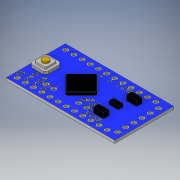
# Autodesk Inventor part: Arduino Pro Mini
Saved by Autodesk Inventor 2016 (Build 200138000, 138)
## iProperties
Created: 2015-11-30
Part Number: Arduino Pro Mini
Material: Generic
Document SubType Name: Modeling
Designer: Spooner
Density: 1 g/cm^3
Appearance: Default
Author: Spooner
Autodesk Inventor part; units mm, degrees
(part 1 of 2)
ref_plane "YZ Plane" through (0, 0, 0) normal (1, 0, 0) x (0, 1, 0)
ref_plane "XZ Plane" through (0, 0, 0) normal (0, 1, 0) x (-1, 0, 0)
sketch "Sketch1" plane through (0, 0, 0) normal (0, 1, 0) x (-1, 0, 0)
  line L0 (0, 0) -> (-33.6804, 0)
  line L1 (-33.6804, 0) -> (-33.6804, -18.3515)
  line L2 (-33.6804, -18.3515) -> (0, -18.3515)
  line L3 (0, -18.3515) -> (0, 0)
  dimension "d0" = 18.3515
  dimension "d1" = 33.6804
  constraints: 8 end point, 2 parallel, 1 horizontal, 1 perpendicular
  measures "d0" distance of L2.end L0.start
  measures "d1" distance of L0.start L0.end
extrude "Extrusion1" add sketch "Sketch1" along normal blind 0.8636
sketch "Sketch2" plane through (0, 0.8636, 0) normal (0, 1, 0) x (1, 0, 0)
  line L0 (14.0415, 4.3942) -> (18.9357, 9.2884)
  line L1 (18.9357, 9.2884) -> (14.0415, 14.1827)
  line L2 (14.0415, 14.1827) -> (9.1472, 9.2884)
  line L3 (9.1472, 9.2884) -> (14.0415, 4.3942)
  line L4 (14.0415, 4.3942) -> (14.0415, 14.1827) construction
  line L5 (18.9357, 9.2884) -> (9.1472, 9.2884) construction
  line L6 (0, 0) -> (33.6804, 0) projected
  line L7 (33.6804, 0) -> (33.6804, 18.3515) projected
  point P0 (14.0415, 9.2884)
  dimension "d4" = 6.9215
  dimension "d5" = 4.3942
  dimension "d6" = 45
  dimension "d7" = 14.7447
  constraints: 12 end point, 2 midpoint, 2 parallel, 2 perpendicular
  measures "d4" distance of L0.end L1.end
  measures "d5" distance from line of L0.start L6
  measures "d6" angle of L6 L0
  measures "d7" distance from line of L0.end L7
extrude "Extrusion2" add sketch "Sketch2" along normal blind 1.1049
chamfer "Chamfer1" distance 0.381 angle 45 4 edges at (14.0415, 1.4161, -4.3942) (18.9357, 1.4161, -9.2884) (14.0415, 1.4161, -14.1827) (9.1472, 1.4161, -9.2884)
chamfer "Chamfer2" distance 0.1905 angle 45 4 edges at (11.5943, 1.9685, -11.7356) (16.4886, 1.9685, -11.7356) (16.4886, 1.9685, -6.8413) (11.5943, 1.9685, -6.8413)
sketch "Sketch3" plane through (0, 0.8636, 0) normal (0, 1, 0) x (1, 0, 0)
  line L0 (0.508, 11.7157) -> (5.588, 11.7157)
  line L1 (5.588, 11.7157) -> (5.588, 6.6357)
  line L2 (5.588, 6.6357) -> (0.508, 6.6357)
  line L3 (0.508, 6.6357) -> (0.508, 11.7157)
  line L4 (0, 18.3515) -> (0, 0) projected
  point P0 (0.508, 9.1758)
  point P1 (0, 9.1758)
  dimension "d16" = 5.08
  dimension "d17" = 0.508
  constraints: 8 end point, 2 midpoint, 2 parallel, 2 perpendicular, 1 horizontal, 1 horizontal alignment
  measures "d16" distance of L0.start L0.end
  measures "d17" distance between parallel lines of L4 L3
extrude "Extrusion3" add sketch "Sketch3" along normal blind 0.889
chamfer "Chamfer3" distance 0.762 angle 45 4 edges at (5.588, 1.3081, -6.6357) (5.588, 1.3081, -11.7157) (0.508, 1.3081, -6.6357) (0.508, 1.3081, -11.7157)
sketch "Sketch4" plane through (0, 1.7526, 0) normal (0, 1, 0) x (1, 0, 0)
  line L0 (0.508, 10.9537) -> (1.27, 11.7157) projected
  line L1 (0.508, 10.9537) -> (0.508, 7.3978) projected
  line L2 (1.27, 6.6357) -> (0.508, 7.3978) projected
  line L3 (1.27, 6.6357) -> (4.826, 6.6357) projected
  line L4 (5.588, 7.3978) -> (4.826, 6.6357) projected
  line L5 (5.588, 7.3978) -> (5.588, 10.9537) projected
  line L6 (4.826, 11.7157) -> (5.588, 10.9537) projected
  line L7 (4.826, 11.7157) -> (1.27, 11.7157) projected
  line L8 (1.5856, 10.9537) -> (1.27, 10.6381)
  line L9 (1.27, 10.6381) -> (1.27, 7.7134)
  line L10 (1.27, 7.7134) -> (1.5856, 7.3978)
  line L11 (1.5856, 7.3978) -> (4.5104, 7.3978)
  line L12 (4.5104, 7.3978) -> (4.826, 7.7134)
  line L13 (4.826, 7.7134) -> (4.826, 10.6381)
  line L14 (4.826, 10.6381) -> (4.5104, 10.9537)
  line L15 (4.5104, 10.9537) -> (1.5856, 10.9537)
  point P0 (0, 0)
  dimension "d23" = 0.762
  constraints: 16 end point, 7 other
  measures "d23" distance between parallel lines of L5 L13
extrude "Extrusion4" add sketch "Sketch4" along normal blind 0.508 draft -5 contours L15 L14 L13 L12 L11 L10 L9 L8
sketch "Sketch5" plane through (0, 2.2606, 0) normal (0, 1, 0) x (1, 0, 0)
  circle A0 centre (3.048, 9.1758) radius 1.016
  line L0 (1.604, 10.9093) -> (4.492, 10.9093) projected
  line L1 (1.3144, 7.7318) -> (1.3144, 10.6197) projected
  point P0 (0, 0)
  point P1 (3.048, 10.9093)
  point P2 (1.3144, 9.1758)
  dimension "d26" = 2.032
  constraints: 2 midpoint, 1 centre point, 1 horizontal alignment, 1 vertical alignment
  measures "d26" diameter of A0
extrude "Extrusion5" add sketch "Sketch5" along normal blind 0.508
sketch "Sketch6" plane through (0, 0.8636, 0) normal (0, 1, 0) x (1, 0, 0)
  line L0 (24.8412, 14.1478) -> (28.0289, 14.1478)
  line L1 (28.0289, 14.1478) -> (28.0289, 12.4841)
  line L2 (28.0289, 12.4841) -> (24.8412, 12.4841)
  line L3 (24.8412, 12.4841) -> (24.8412, 14.1478)
  line L4 (22.9997, 5.7277) -> (26.1874, 5.7277)
  line L5 (26.1874, 5.7277) -> (26.1874, 4.064)
  line L6 (26.1874, 4.064) -> (22.9997, 4.064)
  line L7 (22.9997, 4.064) -> (22.9997, 5.7277)
  line L8 (33.6804, 0) -> (33.6804, 18.3515) projected
  line L9 (0, 0) -> (33.6804, 0) projected
  line L10 (33.6804, 18.3515) -> (0, 18.3515) projected
  dimension "d29" = 3.1877
  dimension "d30" = 1.6637
  dimension "d31" = 5.6515
  dimension "d32" = 7.493
  dimension "d33" = 4.064
  dimension "d34" = 4.2037
  constraints: 16 end point, 6 parallel, 2 horizontal, 2 perpendicular
  measures "d29" distance of L0.start L0.end
  measures "d30" distance of L0.end L1.end
  measures "d31" distance between parallel lines of L8 L1
  measures "d32" distance between parallel lines of L8 L5
  measures "d33" distance between parallel lines of L9 L6
  measures "d34" distance between parallel lines of L10 L0
extrude "Extrusion6" add sketch "Sketch6" along normal blind 1.6129
sketch "Sketch7" plane through (0, 0.8636, 0) normal (0, 1, 0) x (1, 0, 0)
  line L0 (23.1394, 10.2235) -> (26.0604, 10.2235)
  line L1 (26.0604, 10.2235) -> (26.0604, 8.7503)
  line L2 (26.0604, 8.7503) -> (23.1394, 8.7503)
  line L3 (23.1394, 8.7503) -> (23.1394, 10.2235)
  line L4 (33.6804, 0) -> (33.6804, 18.3515) projected
  line L5 (33.6804, 18.3515) -> (0, 18.3515) projected
  point P0 (0, 0)
  dimension "d37" = 2.921
  dimension "d38" = 1.4732
  dimension "d39" = 7.62
  dimension "d40" = 8.128
  constraints: 8 end point, 2 parallel, 1 horizontal, 1 perpendicular
  measures "d37" distance of L0.start L0.end
  measures "d38" distance of L2.end L0.start
  measures "d39" distance between parallel lines of L4 L1
  measures "d40" distance between parallel lines of L5 L0
extrude "Extrusion7" add sketch "Sketch7" along normal blind 1.016
sketch "Sketch8" plane through (0, 0.8636, 0) normal (0, 1, 0) x (1, 0, 0)
  circle A0 centre (1.778, 1.651) radius 0.508
  line L0 (0, 0) -> (33.6804, 0) projected
  line L1 (0, 18.3515) -> (0, 0) projected
  dimension "d43" = 1.016
  dimension "d44" = 1.143
  dimension "d45" = 1.27
  constraints: 1 centre point
  measures "d43" diameter of A0
  measures "d44" distance edge to line of A0 L0
  measures "d45" distance edge to line of A0 L1
extrude "Extrusion8" cut sketch "Sketch8" against normal through all
sketch "Sketch9" plane through (0, 0.8636, 0) normal (0, 1, 0) x (1, 0, 0)
  circle A0 centre (1.778, 1.651) radius 0.508 projected
  circle A1 centre (1.778, 1.651) radius 0.762
  point P0 (0, 0)
  dimension "d48" = 1.524
  constraints: 1 centre point, 1 coincident
  measures "d48" diameter of A1
extrude "Extrusion9" add sketch "Sketch9" along normal blind 0.0254
pattern_linear "Rectangular Pattern1" count 12 spacing 2.54 along (1, 0, 0) of "Extrusion9", "Extrusion8"
sketch "Sketch10" plane through (0, 0.8636, 0) normal (0, 1, 0) x (1, 0, 0)
  circle A0 centre (31.9024, 2.667) radius 0.508
  circle A1 centre (1.778, 1.651) radius 0.508 projected
  line L0 (33.6804, 0) -> (33.6804, 18.3515) projected
  line L1 (0, 0) -> (33.6804, 0) projected
  dimension "d54" = 1.27
  dimension "d55" = 2.159
  constraints: 1 centre point, 1 equal radius
  measures "d54" distance edge to line of A0 L0
  measures "d55" distance edge to line of A0 L1
extrude "Extrusion10" cut sketch "Sketch10" against normal through all contours A0
sketch "Sketch11" plane through (0, 0.8636, 0) normal (0, 1, 0) x (1, 0, 0)
  circle A0 centre (1.778, 1.651) radius 0.762 projected
  circle A1 centre (31.9024, 2.667) radius 0.508 projected
  circle A2 centre (31.9024, 2.667) radius 0.762
  point P0 (0, 0)
  constraints: 1 centre point, 1 coincident, 1 equal radius
extrude "Extrusion11" add sketch "Sketch11" along normal blind 0.0254 contours A2
pattern_linear "Rectangular Pattern2" count 6 spacing 2.54 along (0, 0, -1) of "Extrusion11", "Extrusion10"
ref_plane "Work Plane1" through (0, 0, -9.1758) normal (0, 0, 1) x (1, 0, 0)
mirror "Mirror1" about plane through (0, 0, -9.1758) normal (0, 0, 1) of "Extrusion9", "Extrusion8", "Rectangular Pattern1"
sketch "Sketch12" plane through (0, 0.8636, 0) normal (0, 1, 0) x (1, 0, 0)
  circle A0 centre (7.8232, 4.445) radius 0.508
  circle A1 centre (18.034, 4.445) radius 0.508
  circle A2 centre (1.778, 1.651) radius 0.508 projected
  line L0 (0, 0) -> (33.6804, 0) projected
  line L1 (0, 18.3515) -> (0, 0) projected
  dimension "d63" = 3.937
  dimension "d64" = 7.3152
  dimension "d65" = 17.526
  constraints: 2 centre point, 2 equal radius, 1 horizontal alignment
  measures "d63" distance edge to line of A0 L0
  measures "d64" distance edge to line of A0 L1
  measures "d65" distance edge to line of A1 L1
extrude "Extrusion12" cut sketch "Sketch12" against normal through all contours A0 | A1
sketch "Sketch13" plane through (0, 0.8636, 0) normal (0, 1, 0) x (1, 0, 0)
  circle A0 centre (7.8232, 4.445) radius 0.762
  circle A1 centre (18.034, 4.445) radius 0.762
  circle A2 centre (18.034, 4.445) radius 0.508 projected
  circle A3 centre (7.8232, 4.445) radius 0.508 projected
  circle A4 centre (4.318, 1.651) radius 0.762 projected
  point P0 (0, 0)
  constraints: 2 centre point, 2 concentric, 2 equal radius
extrude "Extrusion13" add sketch "Sketch13" along normal blind 0.0254 contours A0 | A1
pattern_linear "Rectangular Pattern3" count 2 spacing 2.54 along (1, 0, 0) of "Extrusion12", "Extrusion13"
sketch "Sketch14" plane through (0, 0.8636, 0) normal (0, 1, 0) x (1, 0, 0)
  line L0 (0.4732, 2.286) -> (0.4732, 4.4742) construction
  line L1 (0.4732, 4.4742) -> (1.778, 4.4742) construction
  line L2 (1.778, 4.4742) -> (1.778, 2.286) construction
  line L3 (1.778, 2.286) -> (0.4732, 2.286) construction
  line L4 (0, 18.3515) -> (0, 0) projected
  circle A0 centre (1.778, 1.651) radius 0.508 projected
  line L5 (3.0132, 2.286) -> (3.0132, 4.4742) construction
  line L6 (3.0132, 4.4742) -> (4.318, 4.4742) construction
  line L7 (4.318, 4.4742) -> (4.318, 2.286) construction
  line L8 (4.318, 2.286) -> (3.0132, 2.286) construction
  circle A1 centre (4.318, 1.651) radius 0.508 projected
  line L9 (6.858, 2.286) -> (5.5532, 2.286) construction
  line L10 (5.5532, 2.286) -> (5.5532, 4.4742) construction
  line L11 (5.5532, 4.4742) -> (6.858, 4.4742) construction
  line L12 (6.858, 4.4742) -> (6.858, 2.286) construction
  circle A2 centre (6.858, 1.651) radius 0.508 projected
  line L13 (9.398, 2.286) -> (8.0932, 2.286) construction
  line L14 (8.0932, 2.286) -> (8.0932, 4.4742) construction
  line L15 (8.0932, 4.4742) -> (9.398, 4.4742) construction
  line L16 (9.398, 4.4742) -> (9.398, 2.286) construction
  circle A3 centre (9.398, 1.651) radius 0.508 projected
  line L17 (17.1114, 6.0026) -> (18.6587, 7.5499) construction
  line L18 (18.6587, 7.5499) -> (19.5813, 6.6273) construction
  line L19 (19.5813, 6.6273) -> (18.034, 5.08) construction
  line L20 (18.034, 5.08) -> (17.1114, 6.0026) construction
  line L21 (19.6514, 6.0026) -> (21.1987, 7.5499) construction
  line L22 (21.1987, 7.5499) -> (22.1213, 6.6273) construction
  line L23 (22.1213, 6.6273) -> (20.574, 5.08) construction
  line L24 (20.574, 5.08) -> (19.6514, 6.0026) construction
  circle A4 centre (18.034, 4.445) radius 0.508 projected
  circle A5 centre (20.574, 4.445) radius 0.508 projected
  line L25 (14.3109, 4.6636) -> (18.6663, 9.019) projected
  line L26 (22.6916, 2.286) -> (21.3868, 2.286) construction
  line L27 (21.3868, 2.286) -> (21.3868, 4.4742) construction
  line L28 (21.3868, 4.4742) -> (22.6916, 4.4742) construction
  line L29 (22.6916, 4.4742) -> (22.6916, 2.286) construction
  circle A6 centre (22.098, 1.651) radius 0.508 projected
  line L30 (22.905, 3.7002) -> (26.371, 3.7002) construction
  line L31 (26.371, 3.7002) -> (26.371, 2.4138) construction
  line L32 (26.371, 2.4138) -> (22.905, 2.4138) construction
  line L33 (22.905, 2.4138) -> (22.905, 3.7002) construction
  circle A7 centre (24.638, 1.651) radius 0.508 projected
  line L34 (20.365, 16.0655) -> (23.831, 16.0655) construction
  line L35 (23.831, 16.0655) -> (23.831, 14.7791) construction
  line L36 (23.831, 14.7791) -> (20.365, 14.7791) construction
  line L37 (20.365, 14.7791) -> (20.365, 16.0655) construction
  circle A8 centre (22.098, 16.7005) radius 0.508 projected
  circle A9 centre (19.558, 16.7005) radius 0.508 projected
  circle A10 centre (17.018, 16.7005) radius 0.508 projected
  circle A11 centre (14.478, 16.7005) radius 0.508 projected
  line L38 (17.825, 14.7791) -> (17.825, 16.0655) construction
  line L39 (17.825, 16.0655) -> (21.291, 16.0655) construction
  line L40 (21.291, 16.0655) -> (21.291, 14.7791) construction
  line L41 (21.291, 14.7791) -> (17.825, 14.7791) construction
  line L42 (15.4312, 14.7791) -> (15.4312, 16.0655) construction
  line L43 (15.4312, 16.0655) -> (18.6048, 16.0655) construction
  line L44 (18.6048, 16.0655) -> (18.6048, 14.7791) construction
  line L45 (18.6048, 14.7791) -> (15.4312, 14.7791) construction
  line L46 (12.745, 14.7791) -> (12.745, 16.0655) construction
  line L47 (12.745, 16.0655) -> (16.211, 16.0655) construction
  line L48 (16.211, 16.0655) -> (16.211, 14.7791) construction
  line L49 (16.211, 14.7791) -> (12.745, 14.7791) construction
  spline S0 degree 2 poles (1.576, 3.2573) (1.69, 3.1646) (1.778, 2.9877) (1.778, 2.863) knots 0 0 0 1 2 2 2
  spline S1 degree 2 poles (1.778, 2.863) (1.778, 2.6504) (1.5982, 2.516) knots 0 0 0 1 1 1
  spline S2 degree 2 poles (1.5982, 2.516) (1.4165, 2.3778) (1.1227, 2.3778) knots 0 0 0 1 1 1
  spline S3 degree 2 poles (1.1227, 2.3778) (0.798, 2.3778) (0.6278, 2.5334) knots 0 0 0 1 1 1
  spline S4 degree 2 poles (0.6278, 2.5334) (0.4916, 2.6581) (0.4916, 2.8379) knots 0 0 0 1 1 1
  spline S5 degree 2 poles (0.4916, 2.8379) (0.4916, 2.978) (0.5331, 3.0592) knots 0 0 0 1 1 1
  spline S6 degree 2 poles (0.5331, 3.0592) (0.5795, 3.1491) (0.6945, 3.2119) knots 0 0 0 1 1 1
  spline S7 degree 2 poles (0.6945, 3.2119) (0.7187, 3.2255) (0.7409, 3.2255) knots 0 0 0 1 1 1
  spline S8 degree 2 poles (0.7409, 3.2255) (0.7796, 3.2255) (0.8327, 3.1675) (0.8327, 3.1317) knots 0 0 0 1 2 2 2
  spline S9 degree 2 poles (0.8327, 3.1317) (0.8327, 3.0814) (0.7786, 3.0524) knots 0 0 0 1 1 1
  spline S10 degree 2 poles (0.7786, 3.0524) (0.7226, 3.0196) (0.6984, 2.9635) knots 0 0 0 1 1 1
  spline S11 degree 2 poles (0.6984, 2.9635) (0.6781, 2.921) (0.6781, 2.8369) knots 0 0 0 1 1 1
  spline S12 degree 2 poles (0.6781, 2.8369) (0.6781, 2.7277) (0.7757, 2.6523) knots 0 0 0 1 1 1
  spline S13 degree 2 poles (0.7757, 2.6523) (0.8936, 2.5595) (1.1227, 2.5595) knots 0 0 0 1 1 1
  spline S14 degree 2 poles (1.1227, 2.5595) (1.3334, 2.5595) (1.5915, 2.7345) (1.5915, 2.8659) knots 0 0 0 1 2 2 2
  spline S15 degree 2 poles (1.5915, 2.8659) (1.5915, 3.008) (1.4562, 3.1153) knots 0 0 0 1 1 1
  spline S16 degree 2 poles (1.4562, 3.1153) (1.4233, 3.1423) (1.4233, 3.1839) knots 0 0 0 1 1 1
  spline S17 degree 2 poles (1.4233, 3.1839) (1.4233, 3.2197) (1.4803, 3.2796) (1.518, 3.2796) knots 0 0 0 1 2 2 2
  spline S18 degree 2 poles (1.518, 3.2796) (1.5489, 3.2796) (1.576, 3.2573) knots 0 0 0 1 1 1
  spline S19 degree 2 poles (1.4117, 4.3698) (1.778, 4.3698) (1.778, 3.9175) knots 0 0 0 1 1 1
  spline S20 degree 2 poles (1.778, 3.9175) (1.778, 3.6459) (1.5064, 3.499) knots 0 0 0 1 1 1
  spline S21 degree 2 poles (1.5064, 3.499) (1.489, 3.4883) (1.4619, 3.4883) knots 0 0 0 1 1 1
  spline S22 degree 2 poles (1.4619, 3.4883) (1.4214, 3.4883) (1.3585, 3.5483) (1.3585, 3.5869) knots 0 0 0 1 2 2 2
  spline S23 degree 2 poles (1.3585, 3.5869) (1.3585, 3.6333) (1.4011, 3.6517) knots 0 0 0 1 1 1
  spline S24 degree 2 poles (1.4011, 3.6517) (1.5915, 3.7377) (1.5915, 3.9175) knots 0 0 0 1 1 1
  spline S25 degree 2 poles (1.5915, 3.9175) (1.5915, 4.1823) (1.4136, 4.1823) knots 0 0 0 1 1 1
  spline S26 degree 2 poles (1.4136, 4.1823) (1.3257, 4.1823) (1.2561, 4.0161) knots 0 0 0 1 1 1
  spline S27 degree 2 poles (1.2561, 4.0161) (1.1217, 3.6952) (1.1188, 3.6884) knots 0 0 0 1 1 1
  spline S28 degree 2 poles (1.1188, 3.6884) (1.0058, 3.499) (0.8192, 3.499) knots 0 0 0 1 1 1
  spline S29 degree 2 poles (0.8192, 3.499) (0.6452, 3.499) (0.5554, 3.6266) knots 0 0 0 1 1 1
  spline S30 degree 2 poles (0.5554, 3.6266) (0.4848, 3.728) (0.479, 3.8914) knots 0 0 0 1 1 1
  spline S31 degree 2 poles (0.479, 3.8914) (0.4732, 4.0422) (0.5515, 4.1639) knots 0 0 0 1 1 1
  spline S32 degree 2 poles (0.5515, 4.1639) (0.6153, 4.2761) (0.7467, 4.3176) knots 0 0 0 1 1 1
  spline S33 degree 2 poles (0.7467, 4.3176) (0.768, 4.3234) (0.7825, 4.3234) knots 0 0 0 1 1 1
  spline S34 degree 2 poles (0.7825, 4.3234) (0.8212, 4.3234) (0.8685, 4.2664) (0.8685, 4.2297) knots 0 0 0 1 2 2 2
  spline S35 degree 2 poles (0.8685, 4.2297) (0.8685, 4.162) (0.8163, 4.1456) knots 0 0 0 1 1 1
  spline S36 degree 2 poles (0.8163, 4.1456) (0.7371, 4.1204) (0.6578, 3.9822) (0.6617, 3.8981) knots 0 0 0 1 2 2 2
  spline S37 degree 2 poles (0.6617, 3.8981) (0.6704, 3.6807) (0.8154, 3.6807) knots 0 0 0 1 1 1
  spline S38 degree 2 poles (0.8154, 3.6807) (0.8917, 3.6807) (0.9449, 3.757) knots 0 0 0 1 1 1
  spline S39 degree 2 poles (0.9449, 3.757) (0.9855, 3.8141) (1.0348, 3.9503) knots 0 0 0 1 1 1
  spline S40 degree 2 poles (1.0348, 3.9503) (1.1092, 4.1572) (1.1585, 4.2287) knots 0 0 0 1 1 1
  spline S41 degree 2 poles (1.1585, 4.2287) (1.2561, 4.3698) (1.4117, 4.3698) knots 0 0 0 1 1 1
  spline S42 degree 2 poles (4.2155, 3.4178) (4.3093, 3.4178) (4.3093, 3.326) knots 0 0 0 1 1 1
  spline S43 degree 2 poles (4.3093, 3.326) (4.3093, 3.2342) (4.2155, 3.2342) knots 0 0 0 1 1 1
  line L50 (4.2155, 3.2342) -> (3.3621, 3.2342)
  line L51 (3.3621, 3.2342) -> (3.7439, 3.0003)
  spline S44 degree 2 poles (3.7439, 3.0003) (3.8028, 2.9587) (3.8028, 2.8988) knots 0 0 0 1 1 1
  spline S45 degree 2 poles (3.8028, 2.8988) (3.8028, 2.8408) (3.7487, 2.805) knots 0 0 0 1 1 1
  line L52 (3.7487, 2.805) -> (3.3534, 2.5731)
  line L53 (3.3534, 2.5731) -> (4.2155, 2.5731)
  spline S46 degree 2 poles (4.2155, 2.5731) (4.3093, 2.5731) (4.3093, 2.4812) knots 0 0 0 1 1 1
  spline S47 degree 2 poles (4.3093, 2.4812) (4.3093, 2.3875) (4.2155, 2.3875) knots 0 0 0 1 1 1
  line L54 (4.2155, 2.3875) -> (3.1466, 2.3875)
  spline S48 degree 2 poles (3.1466, 2.3875) (3.048, 2.3875) (3.048, 2.487) knots 0 0 0 1 1 1
  spline S49 degree 2 poles (3.048, 2.487) (3.048, 2.5557) (3.1031, 2.5943) knots 0 0 0 1 1 1
  line L55 (3.1031, 2.5943) -> (3.5612, 2.9017)
  line L56 (3.5612, 2.9017) -> (3.1128, 3.2052)
  spline S50 degree 2 poles (3.1128, 3.2052) (3.0393, 3.2564) (3.0393, 3.3221) knots 0 0 0 1 1 1
  spline S51 degree 2 poles (3.0393, 3.3221) (3.0393, 3.3627) (3.1012, 3.4178) (3.1466, 3.4178) knots 0 0 0 1 2 2 2
  line L57 (3.1466, 3.4178) -> (4.2155, 3.4178)
  spline S52 degree 2 poles (3.6801, 4.6491) (3.9353, 4.6491) (4.1015, 4.5293) knots 0 0 0 1 1 1
  spline S53 degree 2 poles (4.1015, 4.5293) (4.318, 4.3891) (4.318, 4.1736) knots 0 0 0 1 1 1
  spline S54 degree 2 poles (4.318, 4.1736) (4.318, 3.9571) (4.1179, 3.8189) knots 0 0 0 1 1 1
  spline S55 degree 2 poles (4.1179, 3.8189) (3.9343, 3.6903) (3.6801, 3.6903) knots 0 0 0 1 1 1
  spline S56 degree 2 poles (3.6801, 3.6903) (3.4259, 3.6903) (3.2394, 3.8112) knots 0 0 0 1 1 1
  spline S57 degree 2 poles (3.2394, 3.8112) (3.0316, 3.9445) (3.0316, 4.1533) knots 0 0 0 1 1 1
  spline S58 degree 2 poles (3.0316, 4.1533) (3.0316, 4.3766) (3.2384, 4.5206) knots 0 0 0 1 1 1
  spline S59 degree 2 poles (3.2384, 4.5206) (3.4259, 4.6491) (3.6801, 4.6491) knots 0 0 0 1 1 1
  spline S60 degree 2 poles (3.6801, 4.4655) (3.4945, 4.4655) (3.3554, 4.3843) knots 0 0 0 1 1 1
  spline S61 degree 2 poles (3.3554, 4.3843) (3.2181, 4.2992) (3.2181, 4.1533) knots 0 0 0 1 1 1
  spline S62 degree 2 poles (3.2181, 4.1533) (3.2181, 4.019) (3.3708, 3.9358) knots 0 0 0 1 1 1
  spline S63 degree 2 poles (3.3708, 3.9358) (3.4897, 3.874) (3.6801, 3.874) knots 0 0 0 1 1 1
  spline S64 degree 2 poles (3.6801, 3.874) (3.8666, 3.874) (3.9836, 3.931) knots 0 0 0 1 1 1
  spline S65 degree 2 poles (3.9836, 3.931) (4.1315, 4.0325) (4.1315, 4.1736) knots 0 0 0 1 1 1
  spline S66 degree 2 poles (4.1315, 4.1736) (4.1315, 4.3128) (3.9836, 4.3998) knots 0 0 0 1 1 1
  spline S67 degree 2 poles (3.9836, 4.3998) (3.8686, 4.4655) (3.6801, 4.4655) knots 0 0 0 1 1 1
  spline S68 degree 2 poles (3.9517, 5.7181) (4.318, 5.7181) (4.318, 5.2658) knots 0 0 0 1 1 1
  spline S69 degree 2 poles (4.318, 5.2658) (4.318, 4.9942) (4.0464, 4.8473) knots 0 0 0 1 1 1
  spline S70 degree 2 poles (4.0464, 4.8473) (4.029, 4.8366) (4.0019, 4.8366) knots 0 0 0 1 1 1
  spline S71 degree 2 poles (4.0019, 4.8366) (3.9614, 4.8366) (3.8985, 4.8966) (3.8985, 4.9352) knots 0 0 0 1 2 2 2
  spline S72 degree 2 poles (3.8985, 4.9352) (3.8985, 4.9816) (3.9411, 5) knots 0 0 0 1 1 1
  spline S73 degree 2 poles (3.9411, 5) (4.1315, 5.086) (4.1315, 5.2658) knots 0 0 0 1 1 1
  spline S74 degree 2 poles (4.1315, 5.2658) (4.1315, 5.5306) (3.9536, 5.5306) knots 0 0 0 1 1 1
  spline S75 degree 2 poles (3.9536, 5.5306) (3.8657, 5.5306) (3.7961, 5.3643) knots 0 0 0 1 1 1
  spline S76 degree 2 poles (3.7961, 5.3643) (3.6617, 5.0435) (3.6588, 5.0367) knots 0 0 0 1 1 1
  spline S77 degree 2 poles (3.6588, 5.0367) (3.5458, 4.8473) (3.3592, 4.8473) knots 0 0 0 1 1 1
  spline S78 degree 2 poles (3.3592, 4.8473) (3.1852, 4.8473) (3.0954, 4.9748) knots 0 0 0 1 1 1
  spline S79 degree 2 poles (3.0954, 4.9748) (3.0248, 5.0763) (3.019, 5.2397) knots 0 0 0 1 1 1
  spline S80 degree 2 poles (3.019, 5.2397) (3.0132, 5.3904) (3.0915, 5.5122) knots 0 0 0 1 1 1
  spline S81 degree 2 poles (3.0915, 5.5122) (3.1553, 5.6243) (3.2867, 5.6659) knots 0 0 0 1 1 1
  spline S82 degree 2 poles (3.2867, 5.6659) (3.308, 5.6717) (3.3225, 5.6717) knots 0 0 0 1 1 1
  spline S83 degree 2 poles (3.3225, 5.6717) (3.3612, 5.6717) (3.4085, 5.6147) (3.4085, 5.5779) knots 0 0 0 1 2 2 2
  spline S84 degree 2 poles (3.4085, 5.5779) (3.4085, 5.5103) (3.3563, 5.4939) knots 0 0 0 1 1 1
  spline S85 degree 2 poles (3.3563, 5.4939) (3.2771, 5.4687) (3.1978, 5.3305) (3.2017, 5.2464) knots 0 0 0 1 2 2 2
  spline S86 degree 2 poles (3.2017, 5.2464) (3.2104, 5.029) (3.3554, 5.029) knots 0 0 0 1 1 1
  spline S87 degree 2 poles (3.3554, 5.029) (3.4317, 5.029) (3.4849, 5.1053) knots 0 0 0 1 1 1
  spline S88 degree 2 poles (3.4849, 5.1053) (3.5255, 5.1623) (3.5748, 5.2986) knots 0 0 0 1 1 1
  spline S89 degree 2 poles (3.5748, 5.2986) (3.6492, 5.5055) (3.6985, 5.577) knots 0 0 0 1 1 1
  spline S90 degree 2 poles (3.6985, 5.577) (3.7961, 5.7181) (3.9517, 5.7181) knots 0 0 0 1 1 1
  spline S91 degree 2 poles (4.2136, 6.1453) (4.3093, 6.1453) (4.3093, 6.0535) knots 0 0 0 1 1 1
  spline S92 degree 2 poles (4.3093, 6.0535) (4.3093, 5.9617) (4.2136, 5.9617) knots 0 0 0 1 1 1
  line L58 (4.2136, 5.9617) -> (3.136, 5.9617)
  spline S93 degree 2 poles (3.136, 5.9617) (3.0432, 5.9617) (3.0432, 6.0535) knots 0 0 0 1 1 1
  spline S94 degree 2 poles (3.0432, 6.0535) (3.0432, 6.1453) (3.136, 6.1453) knots 0 0 0 1 1 1
  line L59 (3.136, 6.1453) -> (4.2136, 6.1453)
  spline S95 degree 2 poles (6.7555, 3.4178) (6.8493, 3.4178) (6.8493, 3.326) knots 0 0 0 1 1 1
  spline S96 degree 2 poles (6.8493, 3.326) (6.8493, 3.2342) (6.7555, 3.2342) knots 0 0 0 1 1 1
  line L60 (6.7555, 3.2342) -> (5.9021, 3.2342)
  line L61 (5.9021, 3.2342) -> (6.2839, 3.0003)
  spline S97 degree 2 poles (6.2839, 3.0003) (6.3428, 2.9587) (6.3428, 2.8988) knots 0 0 0 1 1 1
  spline S98 degree 2 poles (6.3428, 2.8988) (6.3428, 2.8408) (6.2887, 2.805) knots 0 0 0 1 1 1
  line L62 (6.2887, 2.805) -> (5.8934, 2.5731)
  line L63 (5.8934, 2.5731) -> (6.7555, 2.5731)
  spline S99 degree 2 poles (6.7555, 2.5731) (6.8493, 2.5731) (6.8493, 2.4812) knots 0 0 0 1 1 1
  spline S100 degree 2 poles (6.8493, 2.4812) (6.8493, 2.3875) (6.7555, 2.3875) knots 0 0 0 1 1 1
  line L64 (6.7555, 2.3875) -> (5.6866, 2.3875)
  spline S101 degree 2 poles (5.6866, 2.3875) (5.588, 2.3875) (5.588, 2.487) knots 0 0 0 1 1 1
  spline S102 degree 2 poles (5.588, 2.487) (5.588, 2.5557) (5.6431, 2.5943) knots 0 0 0 1 1 1
  line L65 (5.6431, 2.5943) -> (6.1012, 2.9017)
  line L66 (6.1012, 2.9017) -> (5.6528, 3.2052)
  spline S103 degree 2 poles (5.6528, 3.2052) (5.5793, 3.2564) (5.5793, 3.3221) knots 0 0 0 1 1 1
  spline S104 degree 2 poles (5.5793, 3.3221) (5.5793, 3.3627) (5.6412, 3.4178) (5.6866, 3.4178) knots 0 0 0 1 2 2 2
  line L67 (5.6866, 3.4178) -> (6.7555, 3.4178)
  spline S105 degree 2 poles (6.7536, 3.9155) (6.8493, 3.9155) (6.8493, 3.8237) knots 0 0 0 1 1 1
  spline S106 degree 2 poles (6.8493, 3.8237) (6.8493, 3.7319) (6.7536, 3.7319) knots 0 0 0 1 1 1
  line L68 (6.7536, 3.7319) -> (5.676, 3.7319)
  spline S107 degree 2 poles (5.676, 3.7319) (5.5832, 3.7319) (5.5832, 3.8237) knots 0 0 0 1 1 1
  spline S108 degree 2 poles (5.5832, 3.8237) (5.5832, 3.9155) (5.676, 3.9155) knots 0 0 0 1 1 1
  line L69 (5.676, 3.9155) -> (6.7536, 3.9155)
  spline S109 degree 2 poles (6.4917, 5.0986) (6.858, 5.0986) (6.858, 4.6462) knots 0 0 0 1 1 1
  spline S110 degree 2 poles (6.858, 4.6462) (6.858, 4.3746) (6.5864, 4.2277) knots 0 0 0 1 1 1
  spline S111 degree 2 poles (6.5864, 4.2277) (6.569, 4.2171) (6.5419, 4.2171) knots 0 0 0 1 1 1
  spline S112 degree 2 poles (6.5419, 4.2171) (6.5014, 4.2171) (6.4385, 4.277) (6.4385, 4.3157) knots 0 0 0 1 2 2 2
  spline S113 degree 2 poles (6.4385, 4.3157) (6.4385, 4.3621) (6.4811, 4.3804) knots 0 0 0 1 1 1
  spline S114 degree 2 poles (6.4811, 4.3804) (6.6715, 4.4665) (6.6715, 4.6462) knots 0 0 0 1 1 1
  spline S115 degree 2 poles (6.6715, 4.6462) (6.6715, 4.9111) (6.4936, 4.9111) knots 0 0 0 1 1 1
  spline S116 degree 2 poles (6.4936, 4.9111) (6.4057, 4.9111) (6.3361, 4.7448) knots 0 0 0 1 1 1
  spline S117 degree 2 poles (6.3361, 4.7448) (6.2017, 4.4239) (6.1988, 4.4172) knots 0 0 0 1 1 1
  spline S118 degree 2 poles (6.1988, 4.4172) (6.0858, 4.2277) (5.8992, 4.2277) knots 0 0 0 1 1 1
  spline S119 degree 2 poles (5.8992, 4.2277) (5.7252, 4.2277) (5.6354, 4.3553) knots 0 0 0 1 1 1
  spline S120 degree 2 poles (5.6354, 4.3553) (5.5648, 4.4568) (5.559, 4.6201) knots 0 0 0 1 1 1
  spline S121 degree 2 poles (5.559, 4.6201) (5.5532, 4.7709) (5.6315, 4.8927) knots 0 0 0 1 1 1
  spline S122 degree 2 poles (5.6315, 4.8927) (5.6953, 5.0048) (5.8267, 5.0464) knots 0 0 0 1 1 1
  spline S123 degree 2 poles (5.8267, 5.0464) (5.848, 5.0522) (5.8625, 5.0522) knots 0 0 0 1 1 1
  spline S124 degree 2 poles (5.8625, 5.0522) (5.9012, 5.0522) (5.9485, 4.9951) (5.9485, 4.9584) knots 0 0 0 1 2 2 2
  spline S125 degree 2 poles (5.9485, 4.9584) (5.9485, 4.8908) (5.8963, 4.8743) knots 0 0 0 1 1 1
  spline S126 degree 2 poles (5.8963, 4.8743) (5.8171, 4.8492) (5.7378, 4.711) (5.7417, 4.6269) knots 0 0 0 1 2 2 2
  spline S127 degree 2 poles (5.7417, 4.6269) (5.7504, 4.4094) (5.8954, 4.4094) knots 0 0 0 1 1 1
  spline S128 degree 2 poles (5.8954, 4.4094) (5.9717, 4.4094) (6.0249, 4.4858) knots 0 0 0 1 1 1
  spline S129 degree 2 poles (6.0249, 4.4858) (6.0655, 4.5428) (6.1148, 4.6791) knots 0 0 0 1 1 1
  spline S130 degree 2 poles (6.1148, 4.6791) (6.1892, 4.8859) (6.2385, 4.9574) knots 0 0 0 1 1 1
  spline S131 degree 2 poles (6.2385, 4.9574) (6.3361, 5.0986) (6.4917, 5.0986) knots 0 0 0 1 1 1
  spline S132 degree 2 poles (6.2201, 6.2593) (6.4753, 6.2593) (6.6415, 6.1395) knots 0 0 0 1 1 1
  spline S133 degree 2 poles (6.6415, 6.1395) (6.858, 5.9993) (6.858, 5.7838) knots 0 0 0 1 1 1
  spline S134 degree 2 poles (6.858, 5.7838) (6.858, 5.5673) (6.6579, 5.4291) knots 0 0 0 1 1 1
  spline S135 degree 2 poles (6.6579, 5.4291) (6.4743, 5.3006) (6.2201, 5.3006) knots 0 0 0 1 1 1
  spline S136 degree 2 poles (6.2201, 5.3006) (5.9659, 5.3006) (5.7794, 5.4214) knots 0 0 0 1 1 1
  spline S137 degree 2 poles (5.7794, 5.4214) (5.5716, 5.5548) (5.5716, 5.7635) knots 0 0 0 1 1 1
  spline S138 degree 2 poles (5.5716, 5.7635) (5.5716, 5.9868) (5.7784, 6.1308) knots 0 0 0 1 1 1
  spline S139 degree 2 poles (5.7784, 6.1308) (5.9659, 6.2593) (6.2201, 6.2593) knots 0 0 0 1 1 1
  spline S140 degree 2 poles (6.2201, 6.0757) (6.0345, 6.0757) (5.8954, 5.9945) knots 0 0 0 1 1 1
  spline S141 degree 2 poles (5.8954, 5.9945) (5.7581, 5.9095) (5.7581, 5.7635) knots 0 0 0 1 1 1
  spline S142 degree 2 poles (5.7581, 5.7635) (5.7581, 5.6292) (5.9108, 5.5461) knots 0 0 0 1 1 1
  spline S143 degree 2 poles (5.9108, 5.5461) (6.0297, 5.4842) (6.2201, 5.4842) knots 0 0 0 1 1 1
  spline S144 degree 2 poles (6.2201, 5.4842) (6.4066, 5.4842) (6.5236, 5.5412) knots 0 0 0 1 1 1
  spline S145 degree 2 poles (6.5236, 5.5412) (6.6715, 5.6427) (6.6715, 5.7838) knots 0 0 0 1 1 1
  spline S146 degree 2 poles (6.6715, 5.7838) (6.6715, 5.923) (6.5236, 6.01) knots 0 0 0 1 1 1
  spline S147 degree 2 poles (6.5236, 6.01) (6.4086, 6.0757) (6.2201, 6.0757) knots 0 0 0 1 1 1
  spline S148 degree 2 poles (9.0317, 3.2419) (9.398, 3.2419) (9.398, 2.7896) knots 0 0 0 1 1 1
  spline S149 degree 2 poles (9.398, 2.7896) (9.398, 2.518) (9.1264, 2.3711) knots 0 0 0 1 1 1
  spline S150 degree 2 poles (9.1264, 2.3711) (9.109, 2.3604) (9.0819, 2.3604) knots 0 0 0 1 1 1
  spline S151 degree 2 poles (9.0819, 2.3604) (9.0414, 2.3604) (8.9785, 2.4203) (8.9785, 2.459) knots 0 0 0 1 2 2 2
  spline S152 degree 2 poles (8.9785, 2.459) (8.9785, 2.5054) (9.0211, 2.5238) knots 0 0 0 1 1 1
  spline S153 degree 2 poles (9.0211, 2.5238) (9.2115, 2.6098) (9.2115, 2.7896) knots 0 0 0 1 1 1
  spline S154 degree 2 poles (9.2115, 2.7896) (9.2115, 3.0544) (9.0336, 3.0544) knots 0 0 0 1 1 1
  spline S155 degree 2 poles (9.0336, 3.0544) (8.9457, 3.0544) (8.8761, 2.8881) knots 0 0 0 1 1 1
  spline S156 degree 2 poles (8.8761, 2.8881) (8.7417, 2.5673) (8.7388, 2.5605) knots 0 0 0 1 1 1
  spline S157 degree 2 poles (8.7388, 2.5605) (8.6258, 2.3711) (8.4392, 2.3711) knots 0 0 0 1 1 1
  spline S158 degree 2 poles (8.4392, 2.3711) (8.2652, 2.3711) (8.1754, 2.4986) knots 0 0 0 1 1 1
  spline S159 degree 2 poles (8.1754, 2.4986) (8.1048, 2.6001) (8.099, 2.7635) knots 0 0 0 1 1 1
  spline S160 degree 2 poles (8.099, 2.7635) (8.0932, 2.9142) (8.1715, 3.036) knots 0 0 0 1 1 1
  spline S161 degree 2 poles (8.1715, 3.036) (8.2353, 3.1481) (8.3667, 3.1897) knots 0 0 0 1 1 1
  spline S162 degree 2 poles (8.3667, 3.1897) (8.388, 3.1955) (8.4025, 3.1955) knots 0 0 0 1 1 1
  spline S163 degree 2 poles (8.4025, 3.1955) (8.4412, 3.1955) (8.4885, 3.1385) (8.4885, 3.1017) knots 0 0 0 1 2 2 2
  spline S164 degree 2 poles (8.4885, 3.1017) (8.4885, 3.0341) (8.4363, 3.0177) knots 0 0 0 1 1 1
  spline S165 degree 2 poles (8.4363, 3.0177) (8.3571, 2.9925) (8.2778, 2.8543) (8.2817, 2.7702) knots 0 0 0 1 2 2 2
  spline S166 degree 2 poles (8.2817, 2.7702) (8.2904, 2.5528) (8.4354, 2.5528) knots 0 0 0 1 1 1
  spline S167 degree 2 poles (8.4354, 2.5528) (8.5117, 2.5528) (8.5649, 2.6291) knots 0 0 0 1 1 1
  spline S168 degree 2 poles (8.5649, 2.6291) (8.6055, 2.6861) (8.6548, 2.8224) knots 0 0 0 1 1 1
  spline S169 degree 2 poles (8.6548, 2.8224) (8.7292, 3.0292) (8.7785, 3.1008) knots 0 0 0 1 1 1
  spline S170 degree 2 poles (8.7785, 3.1008) (8.8761, 3.2419) (9.0317, 3.2419) knots 0 0 0 1 1 1
  spline S171 degree 2 poles (9.196, 4.3176) (9.31, 4.2248) (9.398, 4.048) (9.398, 3.9233) knots 0 0 0 1 2 2 2
  spline S172 degree 2 poles (9.398, 3.9233) (9.398, 3.7106) (9.2182, 3.5763) knots 0 0 0 1 1 1
  spline S173 degree 2 poles (9.2182, 3.5763) (9.0365, 3.4381) (8.7427, 3.4381) knots 0 0 0 1 1 1
  spline S174 degree 2 poles (8.7427, 3.4381) (8.418, 3.4381) (8.2478, 3.5937) knots 0 0 0 1 1 1
  spline S175 degree 2 poles (8.2478, 3.5937) (8.1116, 3.7184) (8.1116, 3.8981) knots 0 0 0 1 1 1
  spline S176 degree 2 poles (8.1116, 3.8981) (8.1116, 4.0383) (8.1531, 4.1195) knots 0 0 0 1 1 1
  spline S177 degree 2 poles (8.1531, 4.1195) (8.1995, 4.2094) (8.3145, 4.2722) knots 0 0 0 1 1 1
  spline S178 degree 2 poles (8.3145, 4.2722) (8.3387, 4.2857) (8.3609, 4.2857) knots 0 0 0 1 1 1
  spline S179 degree 2 poles (8.3609, 4.2857) (8.3996, 4.2857) (8.4527, 4.2277) (8.4527, 4.192) knots 0 0 0 1 2 2 2
  spline S180 degree 2 poles (8.4527, 4.192) (8.4527, 4.1417) (8.3986, 4.1127) knots 0 0 0 1 1 1
  spline S181 degree 2 poles (8.3986, 4.1127) (8.3426, 4.0799) (8.3184, 4.0238) knots 0 0 0 1 1 1
  spline S182 degree 2 poles (8.3184, 4.0238) (8.2981, 3.9813) (8.2981, 3.8972) knots 0 0 0 1 1 1
  spline S183 degree 2 poles (8.2981, 3.8972) (8.2981, 3.788) (8.3957, 3.7126) knots 0 0 0 1 1 1
  spline S184 degree 2 poles (8.3957, 3.7126) (8.5136, 3.6198) (8.7427, 3.6198) knots 0 0 0 1 1 1
  spline S185 degree 2 poles (8.7427, 3.6198) (8.9534, 3.6198) (9.2115, 3.7947) (9.2115, 3.9262) knots 0 0 0 1 2 2 2
  spline S186 degree 2 poles (9.2115, 3.9262) (9.2115, 4.0683) (9.0762, 4.1755) knots 0 0 0 1 1 1
  spline S187 degree 2 poles (9.0762, 4.1755) (9.0433, 4.2026) (9.0433, 4.2442) knots 0 0 0 1 1 1
  spline S188 degree 2 poles (9.0433, 4.2442) (9.0433, 4.2799) (9.1003, 4.3398) (9.138, 4.3398) knots 0 0 0 1 2 2 2
  spline S189 degree 2 poles (9.138, 4.3398) (9.1689, 4.3398) (9.196, 4.3176) knots 0 0 0 1 1 1
  spline S190 degree 2 poles (9.2617, 5.4233) (9.2704, 5.4339) (9.2936, 5.4339) knots 0 0 0 1 1 1
  spline S191 degree 2 poles (9.2936, 5.4339) (9.3323, 5.4339) (9.3874, 5.374) (9.3874, 5.3383) knots 0 0 0 1 2 2 2
  spline S192 degree 2 poles (9.3874, 5.3383) (9.3874, 5.2899) (9.3371, 5.2609) knots 0 0 0 1 1 1
  line L70 (9.3371, 5.2609) -> (8.6683, 4.8859)
  line L71 (8.6683, 4.8859) -> (8.8113, 4.7535)
  line L72 (8.8113, 4.7535) -> (9.2936, 4.7535)
  spline S193 degree 2 poles (9.2936, 4.7535) (9.3874, 4.7535) (9.3874, 4.6636) knots 0 0 0 1 1 1
  spline S194 degree 2 poles (9.3874, 4.6636) (9.3874, 4.5718) (9.2936, 4.5718) knots 0 0 0 1 1 1
  line L73 (9.2936, 4.5718) -> (8.2169, 4.5718)
  spline S195 degree 2 poles (8.2169, 4.5718) (8.1241, 4.5718) (8.1241, 4.6636) knots 0 0 0 1 1 1
  spline S196 degree 2 poles (8.1241, 4.6636) (8.1241, 4.7535) (8.2169, 4.7535) knots 0 0 0 1 1 1
  line L74 (8.2169, 4.7535) -> (8.5842, 4.7535)
  line L75 (8.5842, 4.7535) -> (8.1512, 5.1904)
  spline S197 degree 2 poles (8.1512, 5.1904) (8.1241, 5.2174) (8.1241, 5.2522) knots 0 0 0 1 1 1
  spline S198 degree 2 poles (8.1241, 5.2522) (8.1241, 5.289) (8.1821, 5.3441) (8.2179, 5.3441) knots 0 0 0 1 2 2 2
  spline S199 degree 2 poles (8.2179, 5.3441) (8.2565, 5.3441) (8.2681, 5.318) knots 0 0 0 1 1 1
  line L76 (8.2681, 5.318) -> (8.5513, 5.0125)
  line L77 (8.5513, 5.0125) -> (9.2617, 5.4233)
  spline S200 degree 2 poles (18.4509, 6.0149) (18.7099, 5.7559) (18.3901, 5.4361) knots 0 0 0 1 1 1
  spline S201 degree 2 poles (18.3901, 5.4361) (18.198, 5.244) (17.9021, 5.3322) knots 0 0 0 1 1 1
  spline S202 degree 2 poles (17.9021, 5.3322) (17.8823, 5.337) (17.8631, 5.3561) knots 0 0 0 1 1 1
  spline S203 degree 2 poles (17.8631, 5.3561) (17.8344, 5.3848) (17.8324, 5.4716) (17.8597, 5.4989) knots 0 0 0 1 2 2 2
  spline S204 degree 2 poles (17.8597, 5.4989) (17.8925, 5.5317) (17.9356, 5.5147) knots 0 0 0 1 1 1
  spline S205 degree 2 poles (17.9356, 5.5147) (18.131, 5.4409) (18.2582, 5.568) knots 0 0 0 1 1 1
  spline S206 degree 2 poles (18.2582, 5.568) (18.4454, 5.7552) (18.3197, 5.881) knots 0 0 0 1 1 1
  spline S207 degree 2 poles (18.3197, 5.881) (18.2575, 5.9432) (18.0907, 5.8748) knots 0 0 0 1 1 1
  spline S208 degree 2 poles (18.0907, 5.8748) (17.7688, 5.7429) (17.762, 5.7402) knots 0 0 0 1 1 1
  spline S209 degree 2 poles (17.762, 5.7402) (17.5481, 5.6862) (17.4162, 5.8181) knots 0 0 0 1 1 1
  spline S210 degree 2 poles (17.4162, 5.8181) (17.2932, 5.9411) (17.3198, 6.0949) knots 0 0 0 1 1 1
  spline S211 degree 2 poles (17.3198, 6.0949) (17.3417, 6.2165) (17.4531, 6.3361) knots 0 0 0 1 1 1
  spline S212 degree 2 poles (17.4531, 6.3361) (17.5556, 6.4469) (17.6971, 6.4776) knots 0 0 0 1 1 1
  spline S213 degree 2 poles (17.6971, 6.4776) (17.8215, 6.5118) (17.9438, 6.4482) knots 0 0 0 1 1 1
  spline S214 degree 2 poles (17.9438, 6.4482) (17.9629, 6.4373) (17.9732, 6.427) knots 0 0 0 1 1 1
  spline S215 degree 2 poles (17.9732, 6.427) (18.0005, 6.3997) (17.9937, 6.3259) (17.9677, 6.2999) knots 0 0 0 1 2 2 2
  spline S216 degree 2 poles (17.9677, 6.2999) (17.9199, 6.2521) (17.8713, 6.2774) knots 0 0 0 1 1 1
  spline S217 degree 2 poles (17.8713, 6.2774) (17.7975, 6.3156) (17.6438, 6.274) (17.587, 6.2118) knots 0 0 0 1 2 2 2
  spline S218 degree 2 poles (17.587, 6.2118) (17.4394, 6.0518) (17.5419, 5.9493) knots 0 0 0 1 1 1
  spline S219 degree 2 poles (17.5419, 5.9493) (17.5959, 5.8953) (17.6875, 5.9117) knots 0 0 0 1 1 1
  spline S220 degree 2 poles (17.6875, 5.9117) (17.7565, 5.9234) (17.8877, 5.9849) knots 0 0 0 1 1 1
  spline S221 degree 2 poles (17.8877, 5.9849) (18.0866, 6.0785) (18.1721, 6.0942) knots 0 0 0 1 1 1
  spline S222 degree 2 poles (18.1721, 6.0942) (18.3409, 6.125) (18.4509, 6.0149) knots 0 0 0 1 1 1
  spline S223 degree 2 poles (18.9867, 7.0045) (19.2266, 6.7647) (19.2252, 6.5118) knots 0 0 0 1 1 1
  spline S224 degree 2 poles (19.2252, 6.5118) (19.2252, 6.3068) (19.0762, 6.1578) knots 0 0 0 1 1 1
  line L78 (19.0762, 6.1578) -> (18.8377, 5.9193)
  line L79 (18.8377, 5.9193) -> (17.954, 6.8029)
  line L80 (17.954, 6.8029) -> (18.1919, 7.0408)
  spline S225 degree 2 poles (18.1919, 7.0408) (18.3388, 7.1877) (18.5425, 7.1973) knots 0 0 0 1 1 1
  spline S226 degree 2 poles (18.5425, 7.1973) (18.7837, 7.2075) (18.9867, 7.0045) knots 0 0 0 1 1 1
  spline S227 degree 2 poles (18.8582, 6.8761) (18.7195, 7.0148) (18.5589, 7.0086) knots 0 0 0 1 1 1
  spline S228 degree 2 poles (18.5589, 7.0086) (18.4208, 7.0032) (18.3245, 6.9068) knots 0 0 0 1 1 1
  line L81 (18.3245, 6.9068) -> (18.2158, 6.7981)
  line L82 (18.2158, 6.7981) -> (18.8343, 6.1796)
  line L83 (18.8343, 6.1796) -> (18.9443, 6.2897)
  spline S229 degree 2 poles (18.9443, 6.2897) (19.0427, 6.3881) (19.0482, 6.5138) knots 0 0 0 1 1 1
  spline S230 degree 2 poles (19.0482, 6.5138) (19.0311, 6.7031) (18.8582, 6.8761) knots 0 0 0 1 1 1
  spline S231 degree 2 poles (20.2299, 7.4617) (20.2483, 7.4529) (20.2599, 7.4412) knots 0 0 0 1 1 1
  spline S232 degree 2 poles (20.2599, 7.4412) (20.2879, 7.4132) (20.2811, 7.3367) (20.2558, 7.3114) knots 0 0 0 1 2 2 2
  spline S233 degree 2 poles (20.2558, 7.3114) (20.2114, 7.267) (20.1547, 7.2923) knots 0 0 0 1 1 1
  line L84 (20.1547, 7.2923) -> (19.9859, 7.3668)
  line L85 (19.9859, 7.3668) -> (19.5888, 6.9697)
  line L86 (19.5888, 6.9697) -> (19.6633, 6.8022)
  spline S234 degree 2 poles (19.6633, 6.8022) (19.6893, 6.7448) (19.6462, 6.7018) knots 0 0 0 1 1 1
  spline S235 degree 2 poles (19.6462, 6.7018) (19.6189, 6.6744) (19.543, 6.6697) (19.5157, 6.697) knots 0 0 0 1 2 2 2
  spline S236 degree 2 poles (19.5157, 6.697) (19.5034, 6.7093) (19.4965, 6.7243) knots 0 0 0 1 1 1
  line L87 (19.4965, 6.7243) -> (19.014, 7.7809)
  spline S237 degree 2 poles (19.014, 7.7809) (18.9833, 7.8486) (19.0393, 7.9046) knots 0 0 0 1 1 1
  spline S238 degree 2 poles (19.0393, 7.9046) (19.0967, 7.962) (19.1555, 7.9347) knots 0 0 0 1 1 1
  line L88 (19.1555, 7.9347) -> (20.2299, 7.4617)
  line L89 (19.8095, 7.4542) -> (19.2314, 7.7126)
  line L90 (19.2314, 7.7126) -> (19.5006, 7.1453)
  line L91 (19.5006, 7.1453) -> (19.8095, 7.4542)
  spline S239 degree 2 poles (20.9909, 6.0149) (21.2499, 5.7559) (20.9301, 5.4361) knots 0 0 0 1 1 1
  spline S240 degree 2 poles (20.9301, 5.4361) (20.738, 5.244) (20.4421, 5.3322) knots 0 0 0 1 1 1
  spline S241 degree 2 poles (20.4421, 5.3322) (20.4223, 5.337) (20.4031, 5.3561) knots 0 0 0 1 1 1
  spline S242 degree 2 poles (20.4031, 5.3561) (20.3744, 5.3848) (20.3724, 5.4716) (20.3997, 5.4989) knots 0 0 0 1 2 2 2
  spline S243 degree 2 poles (20.3997, 5.4989) (20.4325, 5.5317) (20.4756, 5.5147) knots 0 0 0 1 1 1
  spline S244 degree 2 poles (20.4756, 5.5147) (20.671, 5.4409) (20.7982, 5.568) knots 0 0 0 1 1 1
  spline S245 degree 2 poles (20.7982, 5.568) (20.9854, 5.7552) (20.8597, 5.881) knots 0 0 0 1 1 1
  spline S246 degree 2 poles (20.8597, 5.881) (20.7975, 5.9432) (20.6307, 5.8748) knots 0 0 0 1 1 1
  spline S247 degree 2 poles (20.6307, 5.8748) (20.3088, 5.7429) (20.302, 5.7402) knots 0 0 0 1 1 1
  spline S248 degree 2 poles (20.302, 5.7402) (20.0881, 5.6862) (19.9562, 5.8181) knots 0 0 0 1 1 1
  spline S249 degree 2 poles (19.9562, 5.8181) (19.8332, 5.9411) (19.8598, 6.0949) knots 0 0 0 1 1 1
  spline S250 degree 2 poles (19.8598, 6.0949) (19.8817, 6.2165) (19.9931, 6.3361) knots 0 0 0 1 1 1
  spline S251 degree 2 poles (19.9931, 6.3361) (20.0956, 6.4469) (20.2371, 6.4776) knots 0 0 0 1 1 1
  spline S252 degree 2 poles (20.2371, 6.4776) (20.3615, 6.5118) (20.4838, 6.4482) knots 0 0 0 1 1 1
  spline S253 degree 2 poles (20.4838, 6.4482) (20.5029, 6.4373) (20.5132, 6.427) knots 0 0 0 1 1 1
  spline S254 degree 2 poles (20.5132, 6.427) (20.5405, 6.3997) (20.5337, 6.3259) (20.5077, 6.2999) knots 0 0 0 1 2 2 2
  spline S255 degree 2 poles (20.5077, 6.2999) (20.4599, 6.2521) (20.4113, 6.2774) knots 0 0 0 1 1 1
  spline S256 degree 2 poles (20.4113, 6.2774) (20.3375, 6.3156) (20.1838, 6.274) (20.127, 6.2118) knots 0 0 0 1 2 2 2
  spline S257 degree 2 poles (20.127, 6.2118) (19.9794, 6.0518) (20.0819, 5.9493) knots 0 0 0 1 1 1
  spline S258 degree 2 poles (20.0819, 5.9493) (20.1359, 5.8953) (20.2275, 5.9117) knots 0 0 0 1 1 1
  spline S259 degree 2 poles (20.2275, 5.9117) (20.2965, 5.9234) (20.4277, 5.9849) knots 0 0 0 1 1 1
  spline S260 degree 2 poles (20.4277, 5.9849) (20.6266, 6.0785) (20.7121, 6.0942) knots 0 0 0 1 1 1
  spline S261 degree 2 poles (20.7121, 6.0942) (20.8809, 6.125) (20.9909, 6.0149) knots 0 0 0 1 1 1
  spline S262 degree 2 poles (21.8677, 6.6594) (21.8828, 6.5132) (21.8199, 6.3259) (21.7317, 6.2377) knots 0 0 0 1 2 2 2
  spline S263 degree 2 poles (21.7317, 6.2377) (21.5814, 6.0874) (21.3593, 6.1195) knots 0 0 0 1 1 1
  spline S264 degree 2 poles (21.3593, 6.1195) (21.133, 6.1502) (20.9253, 6.358) knots 0 0 0 1 1 1
  spline S265 degree 2 poles (20.9253, 6.358) (20.6957, 6.5876) (20.6854, 6.818) knots 0 0 0 1 1 1
  spline S266 degree 2 poles (20.6854, 6.818) (20.6772, 7.0025) (20.8043, 7.1296) knots 0 0 0 1 1 1
  spline S267 degree 2 poles (20.8043, 7.1296) (20.9034, 7.2287) (20.9902, 7.2567) knots 0 0 0 1 1 1
  spline S268 degree 2 poles (20.9902, 7.2567) (21.0866, 7.2875) (21.2123, 7.2506) knots 0 0 0 1 1 1
  spline S269 degree 2 poles (21.2123, 7.2506) (21.239, 7.2431) (21.2547, 7.2273) knots 0 0 0 1 1 1
  spline S270 degree 2 poles (21.2547, 7.2273) (21.282, 7.2) (21.2786, 7.1214) (21.2533, 7.0961) knots 0 0 0 1 2 2 2
  spline S271 degree 2 poles (21.2533, 7.0961) (21.2178, 7.0606) (21.159, 7.0783) knots 0 0 0 1 1 1
  spline S272 degree 2 poles (21.159, 7.0783) (21.0961, 7.0947) (21.0394, 7.0722) knots 0 0 0 1 1 1
  spline S273 degree 2 poles (21.0394, 7.0722) (20.995, 7.0565) (20.9355, 6.997) knots 0 0 0 1 1 1
  spline S274 degree 2 poles (20.9355, 6.997) (20.8583, 6.9198) (20.874, 6.7975) knots 0 0 0 1 1 1
  spline S275 degree 2 poles (20.874, 6.7975) (20.8918, 6.6485) (21.0538, 6.4865) knots 0 0 0 1 1 1
  spline S276 degree 2 poles (21.0538, 6.4865) (21.2028, 6.3375) (21.5089, 6.2787) (21.6019, 6.3717) knots 0 0 0 1 2 2 2
  spline S277 degree 2 poles (21.6019, 6.3717) (21.7023, 6.4721) (21.6825, 6.6437) knots 0 0 0 1 1 1
  spline S278 degree 2 poles (21.6825, 6.6437) (21.6784, 6.6861) (21.7078, 6.7154) knots 0 0 0 1 1 1
  spline S279 degree 2 poles (21.7078, 6.7154) (21.7331, 6.7407) (21.8158, 6.7428) (21.8424, 6.7161) knots 0 0 0 1 2 2 2
  spline S280 degree 2 poles (21.8424, 6.7161) (21.8643, 6.6943) (21.8677, 6.6594) knots 0 0 0 1 1 1
  line L92 (22.707, 7.2458) -> (22.1753, 6.7141)
  line L93 (22.1753, 6.7141) -> (21.3572, 7.5321)
  spline S281 degree 2 poles (21.3572, 7.5321) (21.2902, 7.5991) (21.3552, 7.664) knots 0 0 0 1 1 1
  spline S282 degree 2 poles (21.3552, 7.664) (21.4187, 7.7276) (21.4857, 7.6606) knots 0 0 0 1 1 1
  line L94 (21.4857, 7.6606) -> (22.1732, 6.9731)
  line L95 (22.1732, 6.9731) -> (22.5764, 7.3763)
  spline S283 degree 2 poles (22.5764, 7.3763) (22.6414, 7.4412) (22.7056, 7.377) knots 0 0 0 1 1 1
  spline S284 degree 2 poles (22.7056, 7.377) (22.7719, 7.3107) (22.707, 7.2458) knots 0 0 0 1 1 1
  line L96 (21.5226, 3.2303) -> (22.5993, 2.9268)
  spline S285 degree 2 poles (22.5993, 2.9268) (22.6776, 2.9055) (22.6776, 2.8147) knots 0 0 0 1 1 1
  spline S286 degree 2 poles (22.6776, 2.8147) (22.6776, 2.7229) (22.6022, 2.6997) knots 0 0 0 1 1 1
  line L97 (22.6022, 2.6997) -> (21.5274, 2.3585)
  spline S287 degree 2 poles (21.5274, 2.3585) (21.511, 2.3546) (21.4946, 2.3546) knots 0 0 0 1 1 1
  spline S288 degree 2 poles (21.4946, 2.3546) (21.4569, 2.3546) (21.4057, 2.4107) (21.4057, 2.4484) knots 0 0 0 1 2 2 2
  spline S289 degree 2 poles (21.4057, 2.4484) (21.4057, 2.5122) (21.4926, 2.5334) knots 0 0 0 1 1 1
  line L98 (21.4926, 2.5334) -> (22.377, 2.8128)
  line L99 (22.377, 2.8128) -> (21.4675, 3.0563)
  spline S290 degree 2 poles (21.4675, 3.0563) (21.4057, 3.0727) (21.4057, 3.1375) knots 0 0 0 1 1 1
  spline S291 degree 2 poles (21.4057, 3.1375) (21.4057, 3.1742) (21.4579, 3.2342) (21.4975, 3.2342) knots 0 0 0 1 2 2 2
  spline S292 degree 2 poles (21.4975, 3.2342) (21.511, 3.2342) (21.5226, 3.2303) knots 0 0 0 1 1 1
  spline S293 degree 2 poles (22.4804, 4.3282) (22.5945, 4.2355) (22.6824, 4.0586) (22.6824, 3.9339) knots 0 0 0 1 2 2 2
  spline S294 degree 2 poles (22.6824, 3.9339) (22.6824, 3.7213) (22.5027, 3.5869) knots 0 0 0 1 1 1
  spline S295 degree 2 poles (22.5027, 3.5869) (22.321, 3.4487) (22.0271, 3.4487) knots 0 0 0 1 1 1
  spline S296 degree 2 poles (22.0271, 3.4487) (21.7024, 3.4487) (21.5323, 3.6043) knots 0 0 0 1 1 1
  spline S297 degree 2 poles (21.5323, 3.6043) (21.396, 3.729) (21.396, 3.9088) knots 0 0 0 1 1 1
  spline S298 degree 2 poles (21.396, 3.9088) (21.396, 4.0489) (21.4376, 4.1301) knots 0 0 0 1 1 1
  spline S299 degree 2 poles (21.4376, 4.1301) (21.484, 4.22) (21.599, 4.2828) knots 0 0 0 1 1 1
  spline S300 degree 2 poles (21.599, 4.2828) (21.6231, 4.2964) (21.6454, 4.2964) knots 0 0 0 1 1 1
  spline S301 degree 2 poles (21.6454, 4.2964) (21.684, 4.2964) (21.7372, 4.2384) (21.7372, 4.2026) knots 0 0 0 1 2 2 2
  spline S302 degree 2 poles (21.7372, 4.2026) (21.7372, 4.1523) (21.6831, 4.1233) knots 0 0 0 1 1 1
  spline S303 degree 2 poles (21.6831, 4.1233) (21.627, 4.0905) (21.6028, 4.0344) knots 0 0 0 1 1 1
  spline S304 degree 2 poles (21.6028, 4.0344) (21.5825, 3.9919) (21.5825, 3.9078) knots 0 0 0 1 1 1
  spline S305 degree 2 poles (21.5825, 3.9078) (21.5825, 3.7986) (21.6802, 3.7232) knots 0 0 0 1 1 1
  spline S306 degree 2 poles (21.6802, 3.7232) (21.7981, 3.6304) (22.0271, 3.6304) knots 0 0 0 1 1 1
  spline S307 degree 2 poles (22.0271, 3.6304) (22.2378, 3.6304) (22.4959, 3.8054) (22.4959, 3.9368) knots 0 0 0 1 2 2 2
  spline S308 degree 2 poles (22.4959, 3.9368) (22.4959, 4.0789) (22.3606, 4.1862) knots 0 0 0 1 1 1
  spline S309 degree 2 poles (22.3606, 4.1862) (22.3277, 4.2132) (22.3277, 4.2548) knots 0 0 0 1 1 1
  spline S310 degree 2 poles (22.3277, 4.2548) (22.3277, 4.2906) (22.3847, 4.3505) (22.4224, 4.3505) knots 0 0 0 1 2 2 2
  spline S311 degree 2 poles (22.4224, 4.3505) (22.4534, 4.3505) (22.4804, 4.3282) knots 0 0 0 1 1 1
  spline S312 degree 2 poles (22.4804, 5.4562) (22.5945, 5.3634) (22.6824, 5.1865) (22.6824, 5.0618) knots 0 0 0 1 2 2 2
  spline S313 degree 2 poles (22.6824, 5.0618) (22.6824, 4.8492) (22.5027, 4.7149) knots 0 0 0 1 1 1
  spline S314 degree 2 poles (22.5027, 4.7149) (22.321, 4.5766) (22.0271, 4.5766) knots 0 0 0 1 1 1
  spline S315 degree 2 poles (22.0271, 4.5766) (21.7024, 4.5766) (21.5323, 4.7322) knots 0 0 0 1 1 1
  spline S316 degree 2 poles (21.5323, 4.7322) (21.396, 4.8569) (21.396, 5.0367) knots 0 0 0 1 1 1
  spline S317 degree 2 poles (21.396, 5.0367) (21.396, 5.1768) (21.4376, 5.258) knots 0 0 0 1 1 1
  spline S318 degree 2 poles (21.4376, 5.258) (21.484, 5.3479) (21.599, 5.4107) knots 0 0 0 1 1 1
  spline S319 degree 2 poles (21.599, 5.4107) (21.6231, 5.4243) (21.6454, 5.4243) knots 0 0 0 1 1 1
  spline S320 degree 2 poles (21.6454, 5.4243) (21.684, 5.4243) (21.7372, 5.3663) (21.7372, 5.3305) knots 0 0 0 1 2 2 2
  spline S321 degree 2 poles (21.7372, 5.3305) (21.7372, 5.2803) (21.6831, 5.2513) knots 0 0 0 1 1 1
  spline S322 degree 2 poles (21.6831, 5.2513) (21.627, 5.2184) (21.6028, 5.1623) knots 0 0 0 1 1 1
  spline S323 degree 2 poles (21.6028, 5.1623) (21.5825, 5.1198) (21.5825, 5.0357) knots 0 0 0 1 1 1
  spline S324 degree 2 poles (21.5825, 5.0357) (21.5825, 4.9265) (21.6802, 4.8511) knots 0 0 0 1 1 1
  spline S325 degree 2 poles (21.6802, 4.8511) (21.7981, 4.7583) (22.0271, 4.7583) knots 0 0 0 1 1 1
  spline S326 degree 2 poles (22.0271, 4.7583) (22.2378, 4.7583) (22.4959, 4.9333) (22.4959, 5.0647) knots 0 0 0 1 2 2 2
  spline S327 degree 2 poles (22.4959, 5.0647) (22.4959, 5.2068) (22.3606, 5.3141) knots 0 0 0 1 1 1
  spline S328 degree 2 poles (22.3606, 5.3141) (22.3277, 5.3412) (22.3277, 5.3827) knots 0 0 0 1 1 1
  spline S329 degree 2 poles (22.3277, 5.3827) (22.3277, 5.4185) (22.3847, 5.4784) (22.4224, 5.4784) knots 0 0 0 1 2 2 2
  spline S330 degree 2 poles (22.4224, 5.4784) (22.4534, 5.4784) (22.4804, 5.4562) knots 0 0 0 1 1 1
  spline S331 degree 2 poles (23.8909, 2.8845) (23.8909, 2.6284) (23.7498, 2.5027) knots 0 0 0 1 1 1
  spline S332 degree 2 poles (23.7498, 2.5027) (23.6502, 2.4138) (23.5178, 2.4138) knots 0 0 0 1 1 1